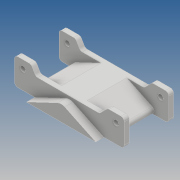
# Autodesk Inventor part: Ball capture zone cover
Saved by Autodesk Inventor 2017 (Build 210142000, 142)
## iProperties
Created: 2017-07-06
Part Number: Ball capture zone cover
Material: Generic
Document SubType Name: Modeling
Designer: yella
Density: 1 g/cm^3
Appearance: Default
Author: yella
Autodesk Inventor part; units mm, degrees
ref_plane "YZ Plane" through (0, 0, 0) normal (1, 0, 0) x (0, 1, 0)
ref_plane "XZ Plane" through (0, 0, 0) normal (0, 1, 0) x (-1, 0, 0)
ref_plane "XY Plane" through (0, 0, 0) normal (0, 0, 1) x (1, 0, 0)
sketch "Sketch1" plane through (0, 0, 0) normal (0, 1, 0) x (-1, 0, 0)
  circle A0 centre (28.2679, -64.7457) radius 1.6
  circle A1 centre (-28.2679, -64.7457) radius 1.6
  line L0 (48.3297, -88.9468) -> (2.1402, -66.9602)
  line L1 (-2.1585, -66.9605) -> (-48.3297, -88.9468)
  arc A2 (2.1402, -66.9602) -> (-2.1585, -66.9605) centre (-0.0088, -71.4748) ccw
  line L2 (28.2679, -64.7457) -> (28.2679, -59.7457)
  line L3 (28.2679, -59.7457) -> (31.2679, -59.7457)
  line L4 (33.2679, -61.7457) -> (33.2679, -73.9415)
  line L5 (-28.2679, -59.7457) -> (-31.2679, -59.7457)
  line L6 (-33.2679, -61.7457) -> (-33.2679, -73.9415)
  line L7 (31.2679, -75.9415) -> (-31.2679, -75.9415)
  line L8 (28.2679, -59.7457) -> (24.4226, -59.7457)
  line L9 (22.6906, -60.7457) -> (20.9585, -63.7457)
  line L10 (-28.2679, -59.7457) -> (-24.0963, -59.7457)
  line L11 (-22.6821, -60.3315) -> (-18.8536, -64.1599)
  line L12 (-17.4394, -64.7457) -> (19.2265, -64.7457)
  arc A3 (24.4226, -59.7457) -> (22.6906, -60.7457) centre (24.4226, -61.7457) ccw
  arc A4 (19.2265, -64.7457) -> (20.9585, -63.7457) centre (19.2265, -62.7457) ccw
  arc A5 (-18.8536, -64.1599) -> (-17.4394, -64.7457) centre (-17.4394, -62.7457) ccw
  arc A6 (-22.6821, -60.3315) -> (-24.0963, -59.7457) centre (-24.0963, -61.7457) ccw
  arc A7 (33.2679, -61.7457) -> (31.2679, -59.7457) centre (31.2679, -61.7457) ccw
  arc A8 (-31.2679, -59.7457) -> (-33.2679, -61.7457) centre (-31.2679, -61.7457) ccw
  arc A9 (31.2679, -75.9415) -> (33.2679, -73.9415) centre (31.2679, -73.9415) ccw
  arc A10 (-33.2679, -73.9415) -> (-31.2679, -75.9415) centre (-31.2679, -73.9415) ccw
  point P0 (0, 0)
  point P1 (33.2679, -59.7457)
  point P2 (-33.2679, -59.7457)
  point P3 (23.2679, -59.7457)
  point P4 (20.3812, -64.7457)
  point P5 (-23.2679, -59.7457)
  dimension "d0" = 3.2
  dimension "d1" = 5
  dimension "d5" = 5
  dimension "d6" = 5
  dimension "d7" = 5
  dimension "d8" = 5
  dimension "d10" = 0
  dimension "d11" = 5
  dimension "d12" = 135
  dimension "d13" = 2
  constraints: 26 end point, 18 point on circle, 18 tangent, 11 centre point, 10 point on line, 7 equal radius, 3 horizontal, 2 perpendicular, 1 parallel, 1 vertical
  measures "d0" diameter of A1
  measures "d1" radius of A2
  measures "d5" distance of L2.start L2.end
  measures "d6" distance of L2.end point (33.268, -59.746)
  measures "d7" distance of L5.start point (-33.268, -59.746)
  measures "d8" distance of L2.end point (23.268, -59.746)
  measures "d10" vertical distance of point (20.381, -64.746) L2.start
  measures "d11" distance of L5.start point (-23.268, -59.746)
  measures "d12" angle of L10 L11
  measures "d13" radius of A3
extrude "Extrusion1" add sketch "Sketch1" along normal blind 3
sketch "Sketch2" plane through (0, 0, 0) normal (0, -1, 0) x (1, 0, 0)
  line L0 (48.3297, -88.9468) -> (2.1402, -66.9602)
  line L1 (-2.1585, -66.9605) -> (-48.3297, -88.9468)
  arc A0 (2.1402, -66.9602) -> (-2.1585, -66.9605) centre (-0.0088, -71.4748) ccw
  line L2 (-31.2679, -75.9415) -> (31.2679, -75.9415) projected
  line L3 (21.008, -75.9415) -> (-21.0185, -75.9415)
  point P0 (0, 0)
  dimension "d16" = 5
  constraints: 6 end point, 4 point on line, 2 point on circle, 2 tangent, 1 centre point
  measures "d16" radius of A0
extrude "Extrusion2" add sketch "Sketch2" along normal blind 5
sketch "Sketch4" plane through (0, 3, 0) normal (0, 1, 0) x (1, 0, 0)
  line L0 (48.3297, -88.9468) -> (2.1402, -66.9602)
  line L1 (-2.1585, -66.9605) -> (-48.3297, -88.9468)
  arc A0 (2.1402, -66.9602) -> (-2.1585, -66.9605) centre (-0.0088, -71.4748) ccw
  line L2 (-21.0185, 75.9415) -> (-2.1585, 66.9605) projected
  arc A1 (-2.1585, 66.9605) -> (2.1402, 66.9602) centre (-0.0088, 71.4748) ccw projected
  line L3 (2.1402, 66.9602) -> (21.008, 75.9415) projected
  line L4 (-31.2679, 75.9415) -> (-21.0185, 75.9415) projected
  line L5 (-31.2679, 75.9415) -> (-7.7569, 64.7457)
  line L6 (-19.2265, 64.7457) -> (17.4394, 64.7457) projected
  arc A2 (33.2679, 73.9415) -> (31.2679, 75.9415) centre (31.2679, 73.9415) ccw projected
  line L7 (21.008, 75.9415) -> (31.2679, 75.9415)
  line L8 (31.2679, 75.9415) -> (7.7478, 64.7457)
  point P0 (0, 0)
  dimension "d21" = 5
  dimension "d22" = 0
  dimension "d23" = 0
  constraints: 10 end point, 3 tangent, 2 point on circle, 2 point on line, 1 centre point, 1 horizontal
  measures "d21" radius of A0
  measures "d22" angle of L5 L2
  measures "d23" angle of L3 L8
extrude "Extrusion4" add sketch "Sketch4" along normal blind 24
sketch "Sketch5" plane through (0, 27, 0) normal (0, 1, 0) x (1, 0, 0)
  line L0 (-7.7569, 64.7457) -> (-31.2679, 75.9415) projected
  arc A0 (-31.2679, 75.9415) -> (-33.2679, 73.9415) centre (-31.2679, 73.9415) ccw projected
  line L1 (-33.2679, 73.9415) -> (-33.2679, 61.7457) projected
  arc A1 (-33.2679, 61.7457) -> (-31.2679, 59.7457) centre (-31.2679, 61.7457) ccw projected
  line L2 (-31.2679, 59.7457) -> (-24.4226, 59.7457) projected
  arc A2 (-24.4226, 59.7457) -> (-22.6906, 60.7457) centre (-24.4226, 61.7457) ccw projected
  line L3 (-22.6906, 60.7457) -> (-20.9585, 63.7457) projected
  arc A3 (-19.2265, 64.7457) -> (-20.9585, 63.7457) centre (-19.2265, 62.7457) ccw projected
  line L4 (-19.2265, 64.7457) -> (-7.7569, 64.7457) projected
  circle A4 centre (-28.2679, 64.7457) radius 1.6 projected
  line L5 (31.2679, 75.9415) -> (7.7478, 64.7457) projected
  line L6 (7.7478, 64.7457) -> (17.4394, 64.7457) projected
  arc A5 (18.8536, 64.1599) -> (17.4394, 64.7457) centre (17.4394, 62.7457) ccw projected
  line L7 (18.8536, 64.1599) -> (22.6821, 60.3315) projected
  arc A6 (22.6821, 60.3315) -> (24.0963, 59.7457) centre (24.0963, 61.7457) ccw projected
  line L8 (24.0963, 59.7457) -> (31.2679, 59.7457) projected
  arc A7 (31.2679, 59.7457) -> (33.2679, 61.7457) centre (31.2679, 61.7457) ccw projected
  line L9 (33.2679, 61.7457) -> (33.2679, 73.9415) projected
  arc A8 (33.2679, 73.9415) -> (31.2679, 75.9415) centre (31.2679, 73.9415) ccw projected
  circle A9 centre (28.2679, 64.7457) radius 1.6 projected
  line L10 (-2.1585, 66.9605) -> (-21.0185, 75.9415) projected
  line L11 (-21.0185, 75.9415) -> (-31.2679, 75.9415) projected
  line L12 (-31.2679, 75.9415) -> (-7.7569, 64.7457) projected
  line L13 (-7.7569, 64.7457) -> (7.7478, 64.7457) projected
  line L14 (7.7478, 64.7457) -> (31.2679, 75.9415) projected
  line L15 (31.2679, 75.9415) -> (21.008, 75.9415) projected
  line L16 (21.008, 75.9415) -> (2.1402, 66.9602) projected
  arc A10 (-2.1585, 66.9605) -> (2.1402, 66.9602) centre (-0.0088, 71.4748) ccw projected
  line L17 (2.1402, 66.9602) -> (21.008, 75.9415) projected
  line L18 (21.008, 75.9415) -> (-21.0185, 75.9415) projected
  line L19 (-21.0185, 75.9415) -> (-2.1585, 66.9605) projected
  arc A11 (-2.1585, 66.9605) -> (2.1402, 66.9602) centre (-0.0088, 71.4748) ccw projected
  point P0 (0, 0)
extrude "Extrusion5" add sketch "Sketch5" along normal blind 3 contours L4 A3 L3 A2 L2 A1 L1 A0 L0 | L0 L11 L10 A10 L16 L15 L5 L13 | L5 A8 L9 A7 L8 A6 L7 A5 L6
fillet "Fillet1" radius 2 2 edges at (-31.2679, 15, -75.9415) (31.2679, 15, -75.9415)
body "Solid1"
